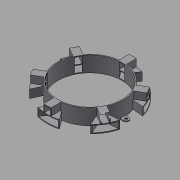
# Autodesk Inventor part: frame3
Saved by Autodesk Inventor 2015 (Build 190159000, 159)
## iProperties
Created: 2016-10-18
Part Number: frame3
Material: Generic
Document SubType Name: Modeling
Designer: Paulo Loma
Density: 1 g/cm^3
Appearance: Default
Author: Paulo Loma
Autodesk Inventor part; units mm, degrees
ref_plane "YZ Plane" through (0, 0, 0) normal (1, 0, 0) x (0, 1, 0)
ref_plane "XZ Plane" through (0, 0, 0) normal (0, 1, 0) x (-1, 0, 0)
ref_plane "XY Plane" through (0, 0, 0) normal (0, 0, 1) x (1, 0, 0)
sketch "Sketch1" plane through (0, 0, 0) normal (0, 0, 1) x (1, 0, 0)
  line L0 (10.6066, 45.6066) -> (2.9972, 34.8714)
  line L1 (-10.6066, 45.6066) -> (-2.9972, 34.8714)
  line L2 (-34.1932, 31.9889) -> (-28.7009, 20.0314)
  line L3 (-44.7998, 13.6177) -> (-31.6982, 14.84)
  line L4 (-44.7998, -13.6177) -> (-31.6982, -14.84)
  line L5 (-34.1932, -31.9889) -> (-28.7009, -20.0314)
  line L6 (-10.6066, -45.6066) -> (-2.9972, -34.8714)
  line L7 (10.6066, -45.6066) -> (2.9972, -34.8714)
  line L8 (34.1932, -31.9889) -> (28.7009, -20.0314)
  line L9 (44.7998, -13.6177) -> (31.6982, -14.84)
  line L10 (44.7998, 13.6177) -> (31.6982, 14.84)
  line L11 (34.1932, 31.9889) -> (28.7009, 20.0314)
  arc A0 (-28.7009, -20.0314) -> (-2.9972, -34.8714) centre (0, 0) ccw
  arc A1 (2.9972, -34.8714) -> (28.7009, -20.0314) centre (0, 0) ccw
  arc A2 (31.6982, -14.84) -> (31.6982, 14.84) centre (0, 0) ccw
  arc A3 (28.7009, 20.0314) -> (2.9972, 34.8714) centre (0, 0) ccw
  arc A4 (-2.9972, 34.8714) -> (-28.7009, 20.0314) centre (0, 0) ccw
  arc A5 (-31.6982, 14.84) -> (-31.6982, -14.84) centre (0, 0) ccw
  line L12 (-4.7955, -35.6792) -> (-11.6512, -45.351)
  line L13 (11.6512, -45.351) -> (4.7955, -35.6792)
  arc A6 (4.7955, -35.6792) -> (28.5013, -21.9926) centre (0, 0) ccw
  line L14 (28.5013, -21.9926) -> (33.4495, -32.7657)
  line L15 (45.1007, -12.5853) -> (33.2968, -13.6865)
  arc A7 (33.2968, -13.6865) -> (33.2968, 13.6865) centre (0, 0) ccw
  line L16 (33.2968, 13.6865) -> (45.1007, 12.5853)
  line L17 (33.4495, 32.7657) -> (28.5013, 21.9926)
  arc A8 (28.5013, 21.9926) -> (4.7955, 35.6792) centre (0, 0) ccw
  line L18 (4.7955, 35.6792) -> (11.6512, 45.351)
  line L19 (-11.6512, 45.351) -> (-4.7955, 35.6792)
  arc A9 (-4.7955, 35.6792) -> (-28.5013, 21.9926) centre (0, 0) ccw
  line L20 (-28.5013, 21.9926) -> (-33.4495, 32.7657)
  line L21 (-45.1007, 12.5853) -> (-33.2968, 13.6865)
  arc A10 (-33.2968, 13.6865) -> (-33.2968, -13.6865) centre (0, 0) ccw
  line L22 (-33.2968, -13.6865) -> (-45.1007, -12.5853)
  line L23 (-33.4495, -32.7657) -> (-28.5013, -21.9926)
  arc A11 (-28.5013, -21.9926) -> (-4.7955, -35.6792) centre (0, 0) ccw
  arc A12 (-11.6512, -45.351) -> (-10.6066, -45.6066) centre (0, 0) ccw
  arc A13 (10.6066, -45.6066) -> (11.6512, -45.351) centre (0, 0) ccw
  arc A14 (33.4495, -32.7657) -> (34.1932, -31.9889) centre (0, 0) ccw
  arc A15 (44.7998, -13.6177) -> (45.1007, -12.5853) centre (0, 0) ccw
  arc A16 (45.1007, 12.5853) -> (44.7998, 13.6177) centre (0, 0) ccw
  arc A17 (34.1932, 31.9889) -> (33.4495, 32.7657) centre (0, 0) ccw
  arc A18 (11.6512, 45.351) -> (10.6066, 45.6066) centre (0, 0) ccw
  arc A19 (-10.6066, 45.6066) -> (-11.6512, 45.351) centre (0, 0) ccw
  arc A20 (-33.4495, 32.7657) -> (-34.1932, 31.9889) centre (0, 0) ccw
  arc A21 (-44.7998, 13.6177) -> (-45.1007, 12.5853) centre (0, 0) ccw
  arc A22 (-45.1007, -12.5853) -> (-44.7998, -13.6177) centre (0, 0) ccw
  arc A23 (-34.1932, -31.9889) -> (-33.4495, -32.7657) centre (0, 0) ccw
  dimension "d12" = 360
  constraints: 48 end point, 48 point on circle, 24 centre point, 3 coincident, 1 other
extrude "Extrusion1" add sketch "Sketch1" along normal blind 7
sketch "Sketch2" plane through (0, 0, 7) normal (0, 0, 1) x (1, 0, 0)
  circle A0 centre (0, 0) radius 35
  line L0 (33.2968, 13.6865) -> (45.1007, 12.5853) projected
  line L1 (33.4495, 32.7657) -> (28.5013, 21.9926) projected
  line L2 (45.1007, -12.5853) -> (33.2968, -13.6865) projected
  line L3 (28.5013, -21.9926) -> (33.4495, -32.7657) projected
  line L4 (11.6512, -45.351) -> (4.7955, -35.6792) projected
  line L5 (-4.7955, -35.6792) -> (-11.6512, -45.351) projected
  line L6 (-33.2968, -13.6865) -> (-45.1007, -12.5853) projected
  line L7 (-33.4495, -32.7657) -> (-28.5013, -21.9926) projected
  line L8 (-45.1007, 12.5853) -> (-33.2968, 13.6865) projected
  line L9 (-28.5013, 21.9926) -> (-33.4495, 32.7657) projected
  line L10 (-11.6512, 45.351) -> (-4.7955, 35.6792) projected
  line L11 (4.7955, 35.6792) -> (11.6512, 45.351) projected
  arc A1 (45.1007, 12.5853) -> (33.4495, 32.7657) centre (0, 0) ccw
  arc A2 (33.4495, -32.7657) -> (45.1007, -12.5853) centre (0, 0) ccw
  arc A3 (-11.6512, -45.351) -> (11.6512, -45.351) centre (0, 0) ccw
  arc A4 (4.7955, -35.6792) -> (28.5013, -21.9926) centre (0, 0) ccw
  arc A5 (-28.5013, -21.9926) -> (-4.7955, -35.6792) centre (0, 0) ccw
  arc A6 (-45.1007, -12.5853) -> (-33.4495, -32.7657) centre (0, 0) ccw
  arc A7 (11.6512, 45.351) -> (-11.6512, 45.351) centre (0, 0) ccw
  arc A8 (-33.4495, 32.7657) -> (-45.1007, 12.5853) centre (0, 0) ccw
  arc A9 (28.5013, 21.9926) -> (4.7955, 35.6792) centre (0, 0) ccw
  arc A10 (-4.7955, 35.6792) -> (-28.5013, 21.9926) centre (0, 0) ccw
  arc A11 (-31.6982, 14.84) -> (-31.6982, -14.84) centre (0, 0) ccw projected
  arc A12 (-33.2968, 13.6865) -> (-33.2968, -13.6865) centre (0, 0) ccw projected
  arc A13 (33.2968, -13.6865) -> (33.2968, 13.6865) centre (0, 0) ccw projected
  point P0 (-10.6066, 45.6066)
  constraints: 24 end point, 21 point on circle, 11 centre point, 3 coincident
extrude "Extrusion2" add sketch "Sketch2" along normal blind 1
sketch "Sketch3" plane through (0, 0, 0) normal (0, 0, -1) x (-1, 0, 0)
  circle A0 centre (0, 0) radius 35
  line L0 (-45.1007, 12.5853) -> (-33.2968, 13.6865) projected
  line L1 (-33.2968, -13.6865) -> (-45.1007, -12.5853) projected
  line L2 (-33.4495, -32.7657) -> (-28.5013, -21.9926) projected
  line L3 (-4.7955, -35.6792) -> (-11.6512, -45.351) projected
  line L4 (11.6512, -45.351) -> (4.7955, -35.6792) projected
  line L5 (28.5013, -21.9926) -> (33.4495, -32.7657) projected
  line L6 (45.1007, -12.5853) -> (33.2968, -13.6865) projected
  line L7 (33.2968, 13.6865) -> (45.1007, 12.5853) projected
  line L8 (33.4495, 32.7657) -> (28.5013, 21.9926) projected
  line L9 (4.7955, 35.6792) -> (11.6512, 45.351) projected
  line L10 (-4.7955, 35.6792) -> (-11.6512, 45.351) projected
  line L11 (-33.4495, 32.7657) -> (-28.5013, 21.9926) projected
  arc A1 (-45.1007, -12.5853) -> (-33.4495, -32.7657) centre (0, 0) ccw
  arc A2 (-28.5013, -21.9926) -> (-4.7955, -35.6792) centre (0, 0) ccw
  arc A3 (-11.6512, -45.351) -> (11.6512, -45.351) centre (0, 0) ccw
  arc A4 (4.7955, -35.6792) -> (28.5013, -21.9926) centre (0, 0) ccw
  arc A5 (33.4495, -32.7657) -> (45.1007, -12.5853) centre (0, 0) ccw
  arc A6 (45.1007, 12.5853) -> (33.4495, 32.7657) centre (0, 0) ccw
  arc A7 (28.5013, 21.9926) -> (4.7955, 35.6792) centre (0, 0) ccw
  arc A8 (-4.7955, 35.6792) -> (-28.5013, 21.9926) centre (0, 0) ccw
  arc A9 (11.6512, 45.351) -> (-11.6512, 45.351) centre (0, 0) ccw
  arc A10 (-33.4495, 32.7657) -> (-45.1007, 12.5853) centre (0, 0) ccw
  arc A11 (33.2968, -13.6865) -> (35.8746, -3.0024) centre (0, 0) ccw
  arc A12 (35.8748, 3) -> (33.2968, 13.6865) centre (0, 0) ccw
  arc A13 (-33.2968, 13.6865) -> (-35.8748, 3) centre (0, 0) ccw
  arc A14 (-35.8748, -3) -> (-33.2968, -13.6865) centre (0, 0) ccw
  circle A15 centre (-39.5, 0) radius 1.5 projected
  arc A16 (-39.5, 3) -> (-39.5, -3) centre (-39.5, 0) ccw projected
  line L12 (-39.5, 3) -> (-35.8748, 3) projected
  line L13 (-35.8748, -3) -> (-39.5, -3) projected
  circle A17 centre (39.5, 0) radius 1.5
  arc A18 (39.5, -3) -> (39.5, 3) centre (39.5, 0) ccw
  line L14 (39.5, -3) -> (35.8748, -3)
  line L15 (35.8748, 3) -> (39.5, 3)
  arc A19 (35.8746, -3.0024) -> (35.8748, -3) centre (0, 0) ccw
  arc A20 (33.2968, -13.6865) -> (35.8748, -3) centre (0, 0) ccw
  arc A21 (4.7955, -35.6792) -> (28.5013, -21.9926) centre (0, 0) ccw
  arc A22 (-35.8748, -3) -> (-33.2968, -13.6865) centre (0, 0) ccw
  arc A23 (-28.5013, -21.9926) -> (-4.7955, -35.6792) centre (0, 0) ccw
  point P0 (-34.1932, 31.9889)
  constraints: 41 point on circle, 28 end point, 22 centre point, 4 coincident, 4 point on line
sketch "Sketch4" plane through (0, 0, 8) normal (0, 0, 1) x (1, 0, 0)
  line L0 (-3.9963, 46.6529) -> (-3.9937, 35.7778)
  line L1 (3.9963, 46.6529) -> (3.9937, 35.7778)
  line L2 (-2.9972, 34.8714) -> (-2.9972, 46.7277)
  line L3 (2.9972, 34.8714) -> (2.9972, 46.7277)
  arc A0 (3.9963, 46.6529) -> (2.9972, 46.7277) centre (0, 0) ccw
  arc A1 (-2.9972, 46.7277) -> (-3.9963, 46.6529) centre (0, 0) ccw
  arc A2 (3.9963, 46.6529) -> (2.9972, 46.7277) centre (0, 0) ccw
  arc A3 (-2.9972, 46.7277) -> (-3.9963, 46.6529) centre (0, 0) ccw
  line L4 (-42.4008, 19.8655) -> (-32.9813, 14.4302)
  line L5 (-38.4044, 26.7874) -> (-28.9876, 21.3475)
  line L6 (-31.6982, 14.84) -> (-41.966, 20.7682)
  line L7 (-28.7009, 20.0314) -> (-38.9688, 25.9595)
  arc A4 (-38.4044, 26.7874) -> (-38.9688, 25.9595) centre (0, 0) ccw
  arc A5 (-41.966, 20.7682) -> (-42.4008, 19.8655) centre (0, 0) ccw
  arc A6 (-38.4044, 26.7874) -> (-38.9688, 25.9595) centre (0, 0) ccw
  arc A7 (-41.966, 20.7682) -> (-42.4008, 19.8655) centre (0, 0) ccw
  line L8 (-38.4044, -26.7874) -> (-28.9876, -21.3475)
  line L9 (-42.4008, -19.8655) -> (-32.9813, -14.4302)
  line L10 (-28.7009, -20.0314) -> (-38.9688, -25.9595)
  line L11 (-31.6982, -14.84) -> (-41.966, -20.7682)
  arc A8 (-42.4008, -19.8655) -> (-41.966, -20.7682) centre (0, 0) ccw
  arc A9 (-38.9688, -25.9595) -> (-38.4044, -26.7874) centre (0, 0) ccw
  arc A10 (-42.4008, -19.8655) -> (-41.966, -20.7682) centre (0, 0) ccw
  arc A11 (-38.9688, -25.9595) -> (-38.4044, -26.7874) centre (0, 0) ccw
  line L12 (3.9963, -46.6529) -> (3.9937, -35.7778)
  line L13 (-3.9963, -46.6529) -> (-3.9937, -35.7778)
  line L14 (2.9972, -34.8714) -> (2.9972, -46.7277)
  line L15 (-2.9972, -34.8714) -> (-2.9972, -46.7277)
  arc A12 (-3.9963, -46.6529) -> (-2.9972, -46.7277) centre (0, 0) ccw
  arc A13 (2.9972, -46.7277) -> (3.9963, -46.6529) centre (0, 0) ccw
  arc A14 (-3.9963, -46.6529) -> (-2.9972, -46.7277) centre (0, 0) ccw
  arc A15 (2.9972, -46.7277) -> (3.9963, -46.6529) centre (0, 0) ccw
  line L16 (42.4008, -19.8655) -> (32.9813, -14.4302)
  line L17 (38.4044, -26.7874) -> (28.9876, -21.3475)
  line L18 (31.6982, -14.84) -> (41.966, -20.7682)
  line L19 (28.7009, -20.0314) -> (38.9688, -25.9595)
  arc A16 (38.4044, -26.7874) -> (38.9688, -25.9595) centre (0, 0) ccw
  arc A17 (41.966, -20.7682) -> (42.4008, -19.8655) centre (0, 0) ccw
  arc A18 (38.4044, -26.7874) -> (38.9688, -25.9595) centre (0, 0) ccw
  arc A19 (41.966, -20.7682) -> (42.4008, -19.8655) centre (0, 0) ccw
  line L20 (38.4044, 26.7874) -> (28.9876, 21.3475)
  line L21 (42.4008, 19.8655) -> (32.9813, 14.4302)
  line L22 (28.7009, 20.0314) -> (38.9688, 25.9595)
  line L23 (31.6982, 14.84) -> (41.966, 20.7682)
  arc A20 (42.4008, 19.8655) -> (41.966, 20.7682) centre (0, 0) ccw
  arc A21 (38.9688, 25.9595) -> (38.4044, 26.7874) centre (0, 0) ccw
  arc A22 (42.4008, 19.8655) -> (41.966, 20.7682) centre (0, 0) ccw
  arc A23 (38.9688, 25.9595) -> (38.4044, 26.7874) centre (0, 0) ccw
  arc A24 (28.7009, 20.0314) -> (2.9972, 34.8714) centre (0, 0) ccw
  arc A25 (28.9876, 21.3475) -> (3.9937, 35.7778) centre (0, 0) ccw
  arc A26 (28.7009, 20.0314) -> (2.9972, 34.8714) centre (0, 0) ccw
  arc A27 (32.9813, -14.4302) -> (32.9813, 14.4302) centre (0, 0) ccw
  arc A28 (31.6982, -14.84) -> (31.6982, 14.84) centre (0, 0) ccw
  arc A29 (31.6982, -14.84) -> (31.6982, 14.84) centre (0, 0) ccw
  arc A30 (2.9972, -34.8714) -> (28.7009, -20.0314) centre (0, 0) ccw
  arc A31 (2.9972, -34.8714) -> (28.7009, -20.0314) centre (0, 0) ccw
  arc A32 (3.9937, -35.7778) -> (28.9876, -21.3475) centre (0, 0) ccw
  arc A33 (-28.9876, -21.3475) -> (-3.9937, -35.7778) centre (0, 0) ccw
  arc A34 (-28.7009, -20.0314) -> (-2.9972, -34.8714) centre (0, 0) ccw
  arc A35 (-28.7009, -20.0314) -> (-2.9972, -34.8714) centre (0, 0) ccw
  arc A36 (-2.9972, 34.8714) -> (-28.7009, 20.0314) centre (0, 0) ccw
  arc A37 (-31.6982, 14.84) -> (-31.6982, -14.84) centre (0, 0) ccw
  arc A38 (-3.9937, 35.7778) -> (-28.9876, 21.3475) centre (0, 0) ccw
  arc A39 (-32.9813, 14.4302) -> (-32.9813, -14.4302) centre (0, 0) ccw
  arc A40 (-2.9972, 34.8714) -> (-28.7009, 20.0314) centre (0, 0) ccw
  arc A41 (-31.6982, 14.84) -> (-31.6982, -14.84) centre (0, 0) ccw
  dimension "d29" = 360
  constraints: 84 point on circle, 48 end point, 42 centre point, 5 coincident, 1 parallel, 1 vertical, 113 other
extrude "Extrusion4" add sketch "Sketch4" along normal blind 7
sketch "Sketch5" plane through (0, 0, 15) normal (0, 0, 1) x (1, 0, 0)
  circle A0 centre (0, 0) radius 35
  line L0 (-38.4044, -26.7874) -> (-28.9876, -21.3475) projected
  line L1 (-32.9813, -14.4302) -> (-42.4008, -19.8655) projected
  line L2 (-3.9937, -35.7778) -> (-3.9963, -46.6529) projected
  line L3 (3.9963, -46.6529) -> (3.9937, -35.7778) projected
  line L4 (28.9876, -21.3475) -> (38.4044, -26.7874) projected
  line L5 (42.4008, -19.8655) -> (32.9813, -14.4302) projected
  line L6 (38.4044, 26.7874) -> (28.9876, 21.3475) projected
  line L7 (32.9813, 14.4302) -> (42.4008, 19.8655) projected
  line L8 (3.9937, 35.7778) -> (3.9963, 46.6529) projected
  line L9 (-3.9963, 46.6529) -> (-3.9937, 35.7778) projected
  line L10 (-28.9876, 21.3475) -> (-38.4044, 26.7874) projected
  line L11 (-42.4008, 19.8655) -> (-32.9813, 14.4302) projected
  arc A1 (-38.4044, 26.7874) -> (-42.4008, 19.8655) centre (0, 0) ccw
  arc A2 (3.9963, 46.6529) -> (-3.9963, 46.6529) centre (0, 0) ccw
  arc A3 (42.4008, 19.8655) -> (38.4044, 26.7874) centre (0, 0) ccw
  arc A4 (38.4044, -26.7874) -> (42.4008, -19.8655) centre (0, 0) ccw
  arc A5 (-42.4008, -19.8655) -> (-38.4044, -26.7874) centre (0, 0) ccw
  arc A6 (-3.9963, -46.6529) -> (3.9963, -46.6529) centre (0, 0) ccw
  arc A7 (3.9937, -35.7778) -> (28.9876, -21.3475) centre (0, 0) ccw
  arc A8 (32.9813, -14.4302) -> (32.9813, 14.4302) centre (0, 0) ccw
  arc A9 (28.9876, 21.3475) -> (3.9937, 35.7778) centre (0, 0) ccw
  arc A10 (-3.9937, 35.7778) -> (-28.9876, 21.3475) centre (0, 0) ccw
  arc A11 (-32.9813, 14.4302) -> (-32.9813, -14.4302) centre (0, 0) ccw
  arc A12 (-28.9876, -21.3475) -> (-3.9937, -35.7778) centre (0, 0) ccw
  constraints: 24 end point, 24 point on circle, 13 centre point, 3 coincident
extrude "Extrusion5" add sketch "Sketch5" along normal blind 1
ref_plane "Work Plane1" through (-44.001, -20.134, -40.4151) normal (0, 0, -1) x (0, 1, 0)
extrude "Extrusion7" add sketch "Sketch3" along normal blind 1
body "Solid1"
